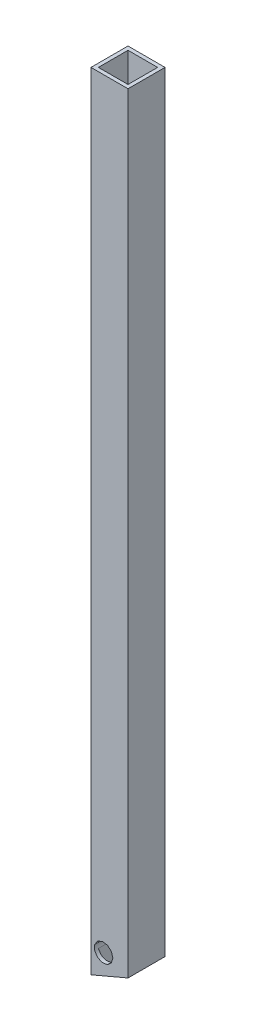
# Autodesk Inventor part: conveyer frame
Saved by Autodesk Inventor 2017 (Build 210142000, 142)
## iProperties
Created: 2020-02-21
Part Number: conveyer frame
Material: Aluminum 6061
Document SubType Name: Sheet Metal
Designer: S346553810
Density: 2.7 g/cm^3
Sheet Metal Rule: Default
Appearance: Aluminum - Flat
Author: S346553810
Autodesk Inventor part; units mm, degrees
ref_plane "YZ Plane" through (0, 0, 0) normal (1, 0, 0) x (0, 1, 0)
ref_plane "XZ Plane" through (0, 0, 0) normal (0, 1, 0) x (-1, 0, 0)
ref_plane "XY Plane" through (0, 0, 0) normal (0, 0, 1) x (1, 0, 0)
sketch "Sketch1" plane through (0, 0, 0) normal (0, 1, 0) x (-1, 0, 0)
  line L0 (12.7, 12.7) -> (-12.7, 12.7)
  line L1 (-12.7, 12.7) -> (-12.7, -12.7)
  line L2 (-12.7, -12.7) -> (12.7, -12.7)
  line L3 (12.7, -12.7) -> (12.7, 12.7)
  line L4 (12.7, 12.7) -> (-12.7, -12.7) construction
  line L5 (-12.7, 12.7) -> (12.7, -12.7) construction
  line L6 (10.16, 10.16) -> (-10.16, 10.16)
  line L7 (-10.16, 10.16) -> (-10.16, -10.16)
  line L8 (-10.16, -10.16) -> (10.16, -10.16)
  line L9 (10.16, -10.16) -> (10.16, 10.16)
  point P0 (0, 0)
  dimension "d0" = 25.4
  dimension "d1" = 25.4
  dimension "d2" = 2.54
  constraints: 20 end point, 4 parallel, 2 midpoint, 2 perpendicular, 1 horizontal, 3 other
  measures "d0" distance of L2.end L1.end
  measures "d1" distance of L1.end L0.end
  measures "d2" distance between parallel lines of L3 L9
extrude "Extrusion1" add sketch "Sketch1" along normal blind 635
sketch "Sketch2" plane through (-12.7, 0, 12.7) normal (0, 0, 1) x (1, 0, 0)
  line L0 (-173.6806, 574.1162) -> (-197.051, 564.1671) construction
  line L1 (-197.051, 564.1671) -> (1.93, 96.7588) construction
  line L2 (25.3004, 106.7078) -> (1.93, 96.7588) construction
  line L3 (-173.6806, 574.1162) -> (25.3004, 106.7078) construction
  line L4 (0, 0) -> (25.4, 0) construction
  line L5 (25.4, 0) -> (25.4, 635)
  line L6 (0, 635) -> (25.4, 635) construction
  line L7 (0, 0) -> (0, 635) construction
  line L8 (-173.6806, 574.1162) -> (-197.051, 564.1671) construction
  line L9 (-197.051, 564.1671) -> (1.93, 96.7588) construction
  line L10 (25.3004, 106.7078) -> (1.93, 96.7588) construction
  line L11 (-173.6806, 574.1162) -> (25.3004, 106.7078) construction
  line L12 (25.4, 0) -> (25.4, 635) construction
  line L13 (0, 0) -> (0, 635) construction
  line L14 (0, 95.9598) -> (0, 0) construction
  line L15 (0, 0) -> (25.4, 0) construction
  line L16 (25.4, 0) -> (25.4, 106.7696) construction
  line L17 (22.86, 0) -> (22.86, 635) construction
  line L18 (25.4, 0) -> (25.4, 635) construction
  line L19 (25.4073, 106.776) -> (0, 95.9598)
  line L20 (0, 0) -> (0, 95.9598)
  line L21 (2.54, 0) -> (2.54, 635) projected
  line L22 (0, 0) -> (25.4, 0)
  line L23 (25.4, 0) -> (25.4073, 106.776)
  line L24 (25.4, 0) -> (25.4073, 0.0057)
  line L25 (25.4073, 0.0057) -> (25.4073, 106.776)
  circle A0 centre (8.6407, 113.4185) radius 6.35 projected
  circle A1 centre (8.6407, 113.4185) radius 6.35 projected
  point P0 (12.7, 0)
  constraints: 18 end point, 4 parallel, 2 point on line, 1 horizontal, 1 vertical
extrude "Extrusion2" cut sketch "Sketch2" against normal blind 128.5875 contours L22 L21 L19 L5 | L5 L19 L23 | L23 L25 L24 | L22 L20 L19 L21
sketch "Sketch4" plane through (-12.7, 635, 12.7) normal (0, 0, 1) x (1, 0, 0)
  circle A0 centre (8.6407, -521.5815) radius 6.35 projected
  point P0 (12.7, -635)
extrude "Extrusion3" cut sketch "Sketch4" against normal blind 128.5875
equation "\"BendRadius\" = Thickness"
equation "\"BendReliefWidth\" = Thickness"
equation "\"BendReliefDepth\" = 0.5 * Thickness"
equation "\"CornerReliefSize\" = 4 * Thickness"
equation "\"MinimumRemnant\" = 2 * Thickness"
equation "\"TransitionRadius\" = BendRadius"
equation "\"JacobiRadiusSize\" = BendRadius"
equation "\"GapSize\" = Thickness"
equation "\"Thickness\" = 3.048"
body "Solid1"
